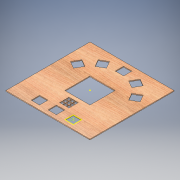
# Autodesk Inventor part: КВ33.045.001 - Основание
Saved by Autodesk Inventor 2019 (Build 230136000, 136)
## iProperties
Created: 2020-02-01
Part Number: КВ33.045.001 - Основание
Material: Дерево (береза)
Document SubType Name: Modeling
Designer: Петров Иван
Density: 0.55 g/cm^3
Appearance: Береза — натуральный — полированный
Author: Петров Иван
Autodesk Inventor part; units mm, degrees
ref_plane "YZ Plane" through (0, 0, 0) normal (1, 0, 0) x (0, 1, 0)
ref_plane "XZ Plane" through (0, 0, 0) normal (0, 1, 0) x (-1, 0, 0)
ref_plane "XY Plane" through (0, 0, 0) normal (0, 0, 1) x (1, 0, 0)
sketch "Эскиз1" plane through (0, 0, 0) normal (0, 1, 0) x (-1, 0, 0)
  line L0 (28, 97) -> (28, 113)
  line L1 (28, 113) -> (12, 113)
  line L2 (12, 113) -> (12, 97)
  line L3 (12, 97) -> (28, 97)
  line L4 (8, 97) -> (8, 113)
  line L5 (8, 113) -> (-8, 113)
  line L6 (-8, 113) -> (-8, 97)
  line L7 (-8, 97) -> (8, 97)
  line L8 (-12, 97) -> (-12, 113)
  line L9 (-12, 113) -> (-28, 113)
  line L10 (-28, 113) -> (-28, 97)
  line L11 (-28, 97) -> (-12, 97)
  line L12 (-12, 117) -> (-12, 133)
  line L13 (-12, 133) -> (-28, 133)
  line L14 (-28, 133) -> (-28, 117)
  line L15 (-28, 117) -> (-12, 117)
  line L16 (8, 133) -> (-8, 133)
  line L17 (-8, 133) -> (-8, 117)
  line L18 (-8, 117) -> (8, 117)
  line L19 (8, 117) -> (8, 133)
  line L20 (28, 117) -> (28, 133)
  line L21 (28, 133) -> (12, 133)
  line L22 (12, 133) -> (12, 117)
  line L23 (12, 117) -> (28, 117)
  line L24 (28, 137) -> (28, 153)
  line L25 (28, 153) -> (12, 153)
  line L26 (12, 153) -> (12, 137)
  line L27 (12, 137) -> (28, 137)
  line L28 (8, 137) -> (8, 153)
  line L29 (8, 153) -> (-8, 153)
  line L30 (-8, 153) -> (-8, 137)
  line L31 (-8, 137) -> (8, 137)
  line L32 (-12, 137) -> (-12, 153)
  line L33 (-12, 153) -> (-28, 153)
  line L34 (-28, 153) -> (-28, 137)
  line L35 (-28, 137) -> (-12, 137)
  line L36 (-75, 225) -> (-125, 225)
  line L37 (-125, 225) -> (-125, 175)
  line L38 (-125, 175) -> (-75, 175)
  line L39 (-75, 175) -> (-75, 225)
  line L40 (25, 225) -> (-25, 225)
  line L41 (-25, 225) -> (-25, 175)
  line L42 (-25, 175) -> (25, 175)
  line L43 (25, 175) -> (25, 225)
  line L44 (125, 225) -> (75, 225)
  line L45 (75, 225) -> (75, 175)
  line L46 (75, 175) -> (125, 175)
  line L47 (125, 175) -> (125, 225)
  line L48 (75, 75) -> (-75, 75)
  line L49 (-75, 75) -> (-75, -75)
  line L50 (-75, -75) -> (75, -75)
  line L51 (75, -75) -> (75, 75)
  line L52 (-139.0544, -109.1506) -> (-164.0544, -65.8494)
  line L53 (-164.0544, -65.8494) -> (-207.3557, -90.8494)
  line L54 (-207.3557, -90.8494) -> (-182.3557, -134.1506)
  line L55 (-182.3557, -134.1506) -> (-139.0544, -109.1506)
  line L56 (-65.8494, -164.0544) -> (-109.1506, -139.0544)
  line L57 (-109.1506, -139.0544) -> (-134.1506, -182.3557)
  line L58 (-134.1506, -182.3557) -> (-90.8494, -207.3557)
  line L59 (-90.8494, -207.3557) -> (-65.8494, -164.0544)
  line L60 (25, -175) -> (-25, -175)
  line L61 (-25, -175) -> (-25, -225)
  line L62 (-25, -225) -> (25, -225)
  line L63 (25, -225) -> (25, -175)
  line L64 (109.1506, -139.0544) -> (65.8494, -164.0544)
  line L65 (65.8494, -164.0544) -> (90.8494, -207.3557)
  line L66 (90.8494, -207.3557) -> (134.1506, -182.3557)
  line L67 (134.1506, -182.3557) -> (109.1506, -139.0544)
  line L68 (164.0544, -65.8494) -> (139.0544, -109.1506)
  line L69 (139.0544, -109.1506) -> (182.3557, -134.1506)
  line L70 (182.3557, -134.1506) -> (207.3557, -90.8494)
  line L71 (207.3557, -90.8494) -> (164.0544, -65.8494)
  line L72 (-250, -250) -> (-250, 250)
  line L73 (-250, 250) -> (250, 250)
  line L74 (250, 250) -> (250, -250)
  line L75 (250, -250) -> (-250, -250)
  line L76 (-75, 225) -> (-125, 225)
  line L77 (-125, 225) -> (-125, 175)
  line L78 (-125, 175) -> (-75, 175)
  line L79 (-75, 175) -> (-75, 225)
  line L80 (28, 153) -> (12, 153)
  line L81 (12, 153) -> (12, 137)
  line L82 (12, 137) -> (28, 137)
  line L83 (28, 137) -> (28, 153)
  line L84 (28, 133) -> (12, 133)
  line L85 (12, 133) -> (12, 117)
  line L86 (12, 117) -> (28, 117)
  line L87 (28, 117) -> (28, 133)
  line L88 (28, 113) -> (12, 113)
  line L89 (12, 113) -> (12, 97)
  line L90 (12, 97) -> (28, 97)
  line L91 (28, 97) -> (28, 113)
  line L92 (8, 113) -> (-8, 113)
  line L93 (-8, 113) -> (-8, 97)
  line L94 (-8, 97) -> (8, 97)
  line L95 (8, 97) -> (8, 113)
  line L96 (-12, 97) -> (-28, 97)
  line L97 (-28, 97) -> (-28, 113)
  line L98 (-28, 113) -> (-12, 113)
  line L99 (-12, 113) -> (-12, 97)
  line L100 (-12, 117) -> (-28, 117)
  line L101 (-28, 117) -> (-28, 133)
  line L102 (-28, 133) -> (-12, 133)
  line L103 (-12, 133) -> (-12, 117)
  line L104 (-12, 137) -> (-28, 137)
  line L105 (-28, 137) -> (-28, 153)
  line L106 (-28, 153) -> (-12, 153)
  line L107 (-12, 153) -> (-12, 137)
  line L108 (8, 153) -> (-8, 153)
  line L109 (-8, 153) -> (-8, 137)
  line L110 (-8, 137) -> (8, 137)
  line L111 (8, 137) -> (8, 153)
  line L112 (8, 133) -> (-8, 133)
  line L113 (-8, 133) -> (-8, 117)
  line L114 (-8, 117) -> (8, 117)
  line L115 (8, 117) -> (8, 133)
  line L116 (75, 75) -> (-75, 75)
  line L117 (-75, 75) -> (-75, -75)
  line L118 (-75, -75) -> (75, -75)
  line L119 (75, -75) -> (75, 75)
  point P0 (0, 0)
  constraints: 240 end point, 22 parallel, 11 horizontal, 11 perpendicular
extrude "Выдавливание1" add sketch "Эскиз1" along normal blind 5
sketch "Эскиз2" plane through (0, 5, 0) normal (0, 1, 0) x (1, 0, 0)
  line L0 (-125, -175) -> (-75, -175) projected
  line L1 (-75, -175) -> (-75, -225) projected
  line L2 (0, 0) -> (-100, -200)
  dimension "d2" = 223.6068
  constraints: 2 end point
  measures "d2" distance of L2.start L2.end
sketch "Эскиз3" plane through (0, 5, 0) normal (0, 1, 0) x (1, 0, 0)
  line L0 (75, -175) -> (125, -175) projected
  line L1 (75, -225) -> (75, -175) projected
  line L2 (125, -225) -> (75, -225) projected
  line L3 (125, -175) -> (125, -225) projected
  point P0 (0, 0)
  point P1 (100, -200)
